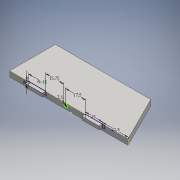
# Autodesk Inventor part: latera_trapezio_agitador
Saved by Autodesk Inventor 2016 (Build 200138000, 138)
## iProperties
Created: 2016-05-23
Part Number: latera_trapezio_agitador
Material: Generic
Document SubType Name: Modeling
Designer: JV
Density: 1 g/cm^3
Appearance: Default
Author: JV
Autodesk Inventor part; units mm, degrees
ref_plane "YZ Plane" through (0, 0, 0) normal (1, 0, 0) x (0, 1, 0)
ref_plane "XZ Plane" through (0, 0, 0) normal (0, 1, 0) x (-1, 0, 0)
ref_plane "XY Plane" through (0, 0, 0) normal (0, 0, 1) x (1, 0, 0)
sketch "Sketch1" plane through (0, 0, 0) normal (0, 0, 1) x (1, 0, 0)
  line L0 (0, -9.797) -> (50, -9.797)
  line L1 (0, -9.797) -> (-50, -9.797)
  line L2 (50, -9.797) -> (30, -9.797)
  line L3 (30, 30.203) -> (50, -9.797)
  line L4 (-50, 30.203) -> (30, 30.203)
  line L5 (-50, -9.797) -> (-54, -9.797)
  line L6 (-50, 30.203) -> (-54, 30.203)
  line L7 (-54, -9.797) -> (-54, 30.203)
  point P0 (0, 0)
  dimension "d4" = 20
  dimension "d5" = 40
  dimension "d27" = 104
  dimension "d29" = 84
  constraints: 16 end point, 5 horizontal, 1 point on line, 1 vertical
  measures "d4" distance of L0.end L2.end
  measures "d5" distance of L2.end L3.start
  measures "d27" distance of L0.end L5.end
  measures "d29" distance of L6.end L3.start
extrude "Extrusion3" add sketch "Sketch1" along normal blind 5
sketch "Sketch3" plane through (-54, -9.797, 0) normal (0, -1, 0) x (1, 0, 0)
  line L0 (104, 0) -> (104, 5) construction
  line L1 (104, 5) -> (81.5, 5) construction
  line L2 (84, 5) -> (0, 5) construction
  line L3 (81.5, 5) -> (66.5, 5)
  line L4 (66.5, 5) -> (66.5, 2)
  line L5 (66.5, 2) -> (81.5, 2)
  line L6 (81.5, 2) -> (81.5, 5)
  line L7 (66.5, 5) -> (66.5, 3) construction
  line L8 (31.5, 2) -> (16.5, 2)
  line L9 (16.5, 2) -> (16.5, 5)
  line L10 (16.5, 5) -> (31.5, 5)
  line L11 (31.5, 5) -> (31.5, 2)
  circle A0 centre (49, 3) radius 1.75
  point P0 (54, 0)
  dimension "d32" = 22.5
  dimension "d33" = 15
  dimension "d34" = 3
  dimension "d41" = 15
  dimension "d42" = 3
  dimension "d44" = 3.5
  dimension "d45" = 15.75
  dimension "d46" = 17.5
  constraints: 20 end point, 4 parallel, 3 point on line, 2 horizontal, 2 perpendicular, 1 centre point
  measures "d32" distance of L0.end L1.end
  measures "d33" distance of L4.end L5.end
  measures "d34" distance of L5.end L1.end
  measures "d41" distance of L8.start L8.end
  measures "d42" distance of L10.end L8.start
  measures "d44" diameter of A0
  measures "d45" distance edge to line of A0 L11
  measures "d46" distance from line of L4 A0.centre
extrude "Extrusion4" add sketch "Sketch3" along normal blind 3 contours L6 L5 L4 L3 | L8 L9 L10 L11
extrude "Extrusion5" cut sketch "Sketch3" against normal blind 15 contours A0
equation "\"d41\" = d33"
equation "\"d42\" = d34"
body "Solid2"
